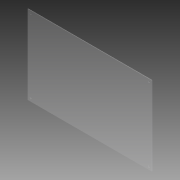
# Autodesk Inventor part: electronics_board
Saved by Autodesk Inventor 2011 (Build 150239000, 239)
## iProperties
Created: 2013-01-19
Part Number: electronics_board
Document SubType Name: Modeling
Designer: Christopher
Density: 1 g/cm^3
Author: Christopher
Autodesk Inventor part; units mm, degrees
ref_plane "YZ Plane" through (0, 0, 0) normal (1, 0, 0) x (0, 1, 0)
ref_plane "XZ Plane" through (0, 0, 0) normal (0, 1, 0) x (-1, 0, 0)
ref_plane "XY Plane" through (0, 0, 0) normal (0, 0, 1) x (1, 0, 0)
sketch "Sketch1" plane through (0, 0, 0) normal (0, 0, 1) x (1, 0, 0)
  line L0 (0, 0) -> (558.8, 0)
  line L1 (558.8, 0) -> (558.8, 355.6)
  line L2 (558.8, 355.6) -> (0, 355.6)
  line L3 (0, 355.6) -> (0, 0)
  dimension "d0" = 558.8
  dimension "d1" = 355.6
  constraints: 8 end point, 2 parallel, 1 horizontal, 1 perpendicular
  measures "d0" distance of L2.end L1.end
  measures "d1" distance of L1.end L0.end
extrude "Extrusion1" add sketch "Sketch1" against normal blind 3.175
sketch "Sketch2" plane through (0, 0, 0) normal (0, 0, 1) x (1, 0, 0)
  line L0 (0, 0) -> (558.8, 0) projected
  line L1 (558.8, 0) -> (558.8, 355.6) projected
  line L2 (558.8, 355.6) -> (0, 355.6) projected
  line L3 (0, 355.6) -> (0, 0) projected
  point P0 (12.7, 342.9)
  point P1 (12.7, 12.7)
  point P2 (546.1, 342.9)
  point P3 (546.1, 12.7)
  dimension "d4" = 12.7
  dimension "d5" = 12.7
  dimension "d6" = 12.7
  dimension "d7" = 12.7
  constraints: 2 horizontal alignment, 2 vertical alignment
  measures "d4" distance from line of L2 point (12.7, 342.9)
  measures "d5" distance from line of L3 point (12.7, 342.9)
  measures "d6" distance from line of L1 point (546.1, 342.9)
  measures "d7" distance from line of L0 point (546.1, 12.7)
hole "Hole1" at (12.7, 342.9, 0) at (12.7, 12.7, 0) at (546.1, 342.9, 0) at (546.1, 12.7, 0) direction (0, 0, -1) diameter 6.35 depth 25.4 tip angle 118
body "Solid1"
